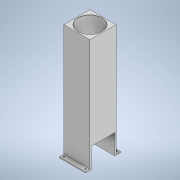
# Autodesk Inventor part: Magazin
Saved by Autodesk Inventor 2020.3 (Build 243373000, 373)
## iProperties
Created: 2021-08-11
Part Number: Magazin
Material: Generisch
Document SubType Name: Modeling
Designer: Preuß P. Ch.
Density: 1 g/cm^3
Appearance: Vorgabe
Author: Preuß P. Ch.
Autodesk Inventor part; units mm, degrees
ref_plane "YZ Plane" through (0, 0, 0) normal (1, 0, 0) x (0, 1, 0)
ref_plane "XZ Plane" through (0, 0, 0) normal (0, 1, 0) x (-1, 0, 0)
ref_plane "XY Plane" through (0, 0, 0) normal (0, 0, 1) x (1, 0, 0)
sketch "Skizze1" plane through (0, 0, 0) normal (0, 1, 0) x (-1, 0, 0)
  line L0 (115, 115) -> (-115, 115)
  line L1 (-115, 115) -> (-115, -115)
  line L2 (-115, -115) -> (115, -115)
  line L3 (115, -115) -> (115, 115)
  point P0 (0, 0)
  dimension "d0" = 230
  dimension "d1" = 230
  constraints: 8 end point, 2 parallel, 1 horizontal, 1 perpendicular
  measures "d0" distance of L2.end L1.end
  measures "d1" distance of L1.end L0.end
extrude "Extrusion1" add sketch "Skizze1" along normal blind 1000
sketch "Skizze2" plane through (115, 0, 115) normal (1, 0, 0) x (0, 0, -1)
  line L0 (0, 0) -> (230, 0) projected
  line L1 (10, 0) -> (220, 0)
  line L2 (220, 0) -> (220, 180)
  line L3 (220, 180) -> (10, 180)
  line L4 (10, 180) -> (10, 0)
  point P0 (115, 0)
  dimension "d4" = 210
  dimension "d5" = 180
  constraints: 8 end point, 2 parallel, 1 horizontal, 1 perpendicular, 1 point on line
  measures "d4" distance of L3.end L2.end
  measures "d5" distance of L2.end L1.end
extrude "Extrusion2" cut sketch "Skizze2" against normal blind 230
sketch "Skizze3" plane through (0, 1000, 0) normal (0, 1, 0) x (1, 0, 0)
  circle A0 centre (0, 0) radius 105
  dimension "d8" = 210
  constraints: 1 centre point, 1 coincident
  measures "d8" diameter of A0
extrude "Extrusion3" cut sketch "Skizze3" against normal blind 820
chamfer "Fase1" distance 2 angle 45 1 edges at (-105, 1000, 0)
sketch "Skizze4" plane through (115, 0, -115) normal (0, 0, -1) x (-1, 0, 0)
  line L0 (230, 0) -> (0, 0) projected
  line L1 (230, 180) -> (230, 0) projected
  line L2 (0, 0) -> (230, 0)
  line L3 (230, 0) -> (230, 10)
  line L4 (230, 10) -> (0, 10)
  line L5 (0, 10) -> (0, 0)
  point P0 (115, 0)
  dimension "d14" = 10
  constraints: 8 end point, 2 parallel, 1 horizontal, 1 perpendicular, 1 point on line
  measures "d14" distance of L3.end L2.end
extrude "Extrusion4" add sketch "Skizze4" along normal blind 40
sketch "Skizze5" plane through (-115, 0, 115) normal (0, 0, 1) x (1, 0, 0)
  line L0 (230, 0) -> (0, 0) projected
  line L1 (230, 180) -> (230, 0) projected
  line L2 (0, 0) -> (230, 0)
  line L3 (230, 0) -> (230, 10)
  line L4 (230, 10) -> (0, 10)
  line L5 (0, 10) -> (0, 0)
  point P0 (115, 0)
  dimension "d17" = 10
  constraints: 8 end point, 2 parallel, 1 horizontal, 1 perpendicular, 1 point on line
  measures "d17" distance of L3.end L2.end
extrude "Extrusion5" add sketch "Skizze5" along normal blind 40
sketch "Skizze6" plane through (-115, 10, 115) normal (0, 1, 0) x (1, 0, 0)
  line L0 (230, -40) -> (0, -40) projected
  line L1 (0, -40) -> (20, -40)
  line L2 (20, -40) -> (20, -20)
  line L3 (20, -20) -> (0, -20)
  line L4 (0, -20) -> (0, -40)
  line L5 (230, 0) -> (230, -40) projected
  line L6 (230, -40) -> (210, -40)
  line L7 (210, -40) -> (210, -20)
  line L8 (210, -20) -> (230, -20)
  line L9 (230, -20) -> (230, -40)
  line L10 (230, 270.1888) -> (210, 270.1888)
  line L11 (210, 270.1888) -> (210, 250.1888)
  line L12 (210, 250.1888) -> (230, 250.1888)
  line L13 (230, 250.1888) -> (230, 270.1888)
  line L14 (0, 270) -> (230, 270) projected
  line L15 (0, 270) -> (20, 270)
  line L16 (20, 270) -> (20, 250)
  line L17 (20, 250) -> (0, 250)
  line L18 (0, 250) -> (0, 270)
  point P0 (115, 115)
  dimension "d20" = 20
  dimension "d21" = 20
  dimension "d22" = 20
  dimension "d23" = 20
  dimension "d24" = 20
  constraints: 32 end point, 8 parallel, 4 horizontal, 4 perpendicular, 4 point on line
  measures "d20" distance of L3.end L2.end
  measures "d21" distance of L2.end L1.end
  measures "d22" distance of L7.end L8.end
  measures "d23" distance of L11.end L10.end
  measures "d24" distance of L15.end L16.end
hole "Bohrung1" at (-95, 10, 135) at (95, 10, 135) at (-95, 10, -135) at (95, 10, -135.1888) direction (0, -1, 0) diameter 10 depth 10 tip angle 118 countersink diameter 14 countersink angle 90
